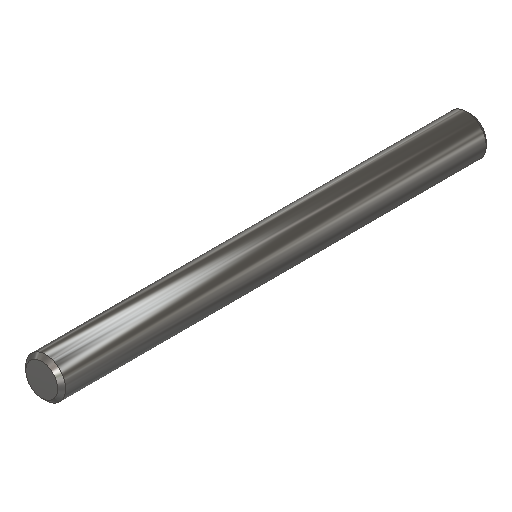
# Autodesk Inventor part: CUT_STEEL_5x53,5_Linear_rod
Saved by Autodesk Inventor 2025 (Build 290162010, 162A)
## iProperties
Created: 2018-06-17
Part Number: CUT_STEEL_5x53,5_Linear_rod
Material: Stainless Steel
Document SubType Name: Modeling
Designer: Andrzej
Density: 8 g/cm^3
Appearance: Steel - Polished
Author: Andrzej
Autodesk Inventor part; units mm, degrees
ref_plane "YZ Plane" through (0, 0, 0) normal (1, 0, 0) x (0, 1, 0)
ref_plane "XZ Plane" through (0, 0, 0) normal (0, 1, 0) x (-1, 0, 0)
ref_plane "XY Plane" through (0, 0, 0) normal (0, 0, 1) x (1, 0, 0)
sketch "Sketch1" plane through (0, 0, 0) normal (0, 0, 1) x (1, 0, 0)
  circle A0 centre (0, 0) radius 2.5
  dimension "d0" = 5
  constraints: 1 centre point, 1 coincident
  measures "d0" diameter of A0
extrude "Extrusion1" add sketch "Sketch1" along normal blind 53.5
chamfer "Chamfer1" distance 0.5 angle 45 2 edges at (-2.5, 0, 0) (-2.5, 0, 53.5)
body "Solid1"
